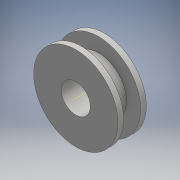
# Autodesk Inventor part: REEL
Saved by Autodesk Inventor 2016 (Build 200138000, 138)
## iProperties
Created: 2016-04-19
Part Number: REEL
Material: Generic
Document SubType Name: Modeling
Designer: Kenneth Daniel
Density: 1 g/cm^3
Appearance: Default
Author: Kenneth Daniel
Autodesk Inventor part; units mm, degrees
ref_plane "YZ Plane" through (0, 0, 0) normal (1, 0, 0) x (0, 1, 0)
ref_plane "XZ Plane" through (0, 0, 0) normal (0, 1, 0) x (-1, 0, 0)
ref_plane "XY Plane" through (0, 0, 0) normal (0, 0, 1) x (1, 0, 0)
sketch "Sketch1" plane through (0, 0, 0) normal (0, 1, 0) x (-1, 0, 0)
  circle A0 centre (0, 0) radius 4.8 construction
  circle A1 centre (0, 0) radius 14.8
  circle A2 centre (0, 0) radius 5.1
  dimension "d0" = 9.6
  dimension "d1" = 10
  dimension "d2" = 0.3
  constraints: 3 centre point, 1 coincident
  measures "d0" diameter of A0
  measures "d1" radial gap between concentric circles of A0 A1
  measures "d2" radial gap between concentric circles of A0 A2
extrude "Extrusion1" add sketch "Sketch1" along normal blind 10
sketch "Sketch2" plane through (0, 0, 0) normal (1, 0, 0) x (0, 1, 0)
  line L0 (10, -14.8) -> (10, 14.8) projected
  line L1 (0, 14.8) -> (0, -14.8) projected
  line L2 (0, 14.8) -> (0, -14.8) projected
  line L3 (0, -14.8) -> (2, -14.8)
  line L4 (0, -14.8) -> (10, -14.8) projected
  line L5 (2, -14.8) -> (2, -9.8)
  line L6 (10, -14.8) -> (8, -14.8)
  line L7 (8, -14.8) -> (8, -9.8)
  line L8 (8, -9.8) -> (2, -9.8)
  line L9 (2, -14.8) -> (8, -14.8)
  line L10 (-2, 0) -> (12, 0) projected
  point P0 (0, 0)
  dimension "d5" = 2
  dimension "d6" = 5
  dimension "d7" = 2
  dimension "d8" = 5
  constraints: 12 end point, 2 perpendicular, 2 point on line, 1 horizontal
  measures "d5" distance of L1.end L3.end
  measures "d6" distance of L3.end L5.end
  measures "d7" distance of L4.end L6.end
  measures "d8" distance of L6.end L7.end
revolve "Revolution1" cut sketch "Sketch2" angle 360 about axis through (0, 0, 0) along (0, 1, 0) contours L4 L5 L8 L7
body "Solid1"
